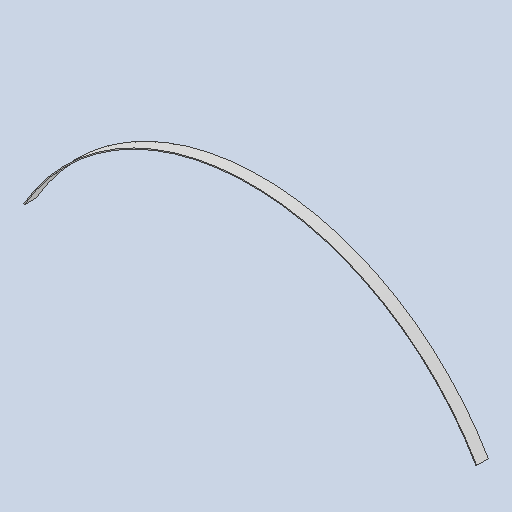
# Autodesk Inventor part: DMF 2.1 01 44 Gear rim 4
Saved by Autodesk Inventor 2025 (Build 290162010, 162A)
## iProperties
Created: 2024-04-30
Part Number: DMF 2.1 01 44 Gear rim 4
Material: Generic
Document SubType Name: Sheet Metal
Designer: admin
Stock Number: Барабан_Сектор_Усилителя
Density: 1 g/cm^3
Flat Pattern Width: 2.5 cm
Flat Pattern Length: 117.052 cm
Flat Pattern Area: 292.629 cm^2
Sheet Metal Rule: Default
Sheet Metal Width: 25,000 mm
Sheet Metal Length: 1170,516 mm
Sheet Metal Area: 29262,888 mm^2
Appearance: Default
Author: pokla
Autodesk Inventor part; units mm, degrees
ref_plane "YZ Plane" through (0, 0, 0) normal (1, 0, 0) x (0, 1, 0)
ref_plane "XZ Plane" through (0, 0, 0) normal (0, 1, 0) x (-1, 0, 0)
ref_plane "XY Plane" through (0, 0, 0) normal (0, 0, 1) x (1, 0, 0)
sketch "Sketch1" plane through (0, 0, 0) normal (0, 0, 1) x (1, 0, 0)
  arc A0 (484.9742, 280) -> (-484.9742, 280) centre (0, 0) ccw
  line L0 (0, 0) -> (-484.9742, 280) construction
  line L1 (0, 0) -> (0, 362.16) construction
  line L2 (0, 0) -> (484.9742, 280) construction
  arc A1 (-484.9742, 280) -> (484.9742, 280) centre (0, 0) ccw construction
  point P0 (-311.7691, 180)
  point P1 (311.7691, 180)
  dimension "d28" = 1120
  dimension "d30" = 120
  measures "d28" diameter of A0
  measures "d30" angle of L2 L0
contour flange "Contour Flange1" sketch "Sketch1" thickness 2 bend radius 2 width 25 along (0, 0, 1) mid plane no both sides no wall seen from (0, 560, 0) lies toward (0, -1, 0) curves A0
bend "Bend1"
corner "Corner1"
equation "\"d28\" = Шстр_диам_внутр"
equation "\"d31\" = Thickness"
equation "\"d32\" = BendReliefWidth"
equation "\"d33\" = BendReliefDepth"
equation "\"d34\" = MinimumRemnant"
equation "\"d35\" = TransitionRadius"
equation "\"d37\" = BendRadius"
equation "\"d39\" = CornerReliefSize"
equation "\"d40\" = GapSize"
equation "\"d41\" = JacobiRadiusSize"
equation "\"BendRadius\" = Thickness"
equation "\"BendReliefWidth\" = Thickness"
equation "\"BendReliefDepth\" = 0.5 * Thickness"
equation "\"CornerReliefSize\" = 4 * Thickness"
equation "\"MinimumRemnant\" = 2 * Thickness"
equation "\"TransitionRadius\" = BendRadius"
equation "\"JacobiRadiusSize\" = BendRadius"
equation "\"GapSize\" = Thickness"
equation "\"Шстр_диам_внутр\" = 1120"
equation "\"Thickness\" = 2"
body "Solid2"
